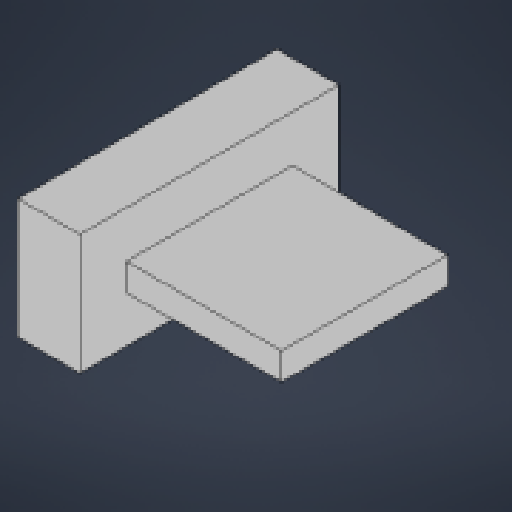
# Autodesk Inventor part: seguro1
Saved by Autodesk Inventor 2026.2 (Build 302298010, 298A)
## iProperties
Created: 2026-08-22
Part Number: seguro1
Material: Genérico
Document SubType Name: Modeling
Designer: samue
Density: 1 g/cm^3
Appearance: Valor por defecto
Author: samue
Autodesk Inventor part; units mm, degrees
ref_plane "YZ Plane" through (0, 0, 0) normal (1, 0, 0) x (0, 1, 0)
ref_plane "XZ Plane" through (0, 0, 0) normal (0, 1, 0) x (-1, 0, 0)
ref_plane "XY Plane" through (0, 0, 0) normal (0, 0, 1) x (1, 0, 0)
sketch "Boceto1" plane through (0, 0, 0) normal (1, 0, 0) x (0, 1, 0)
  line L0 (0, 0) -> (1.75, 0)
  line L1 (1.75, 0) -> (1.75, -10.7)
  line L2 (1.75, -10.7) -> (0, -10.7)
  line L3 (0, -10.7) -> (0, 0)
  dimension "d0" = 1.75
  dimension "d1" = 10.7
  constraints: 8 end point, 2 parallel, 1 horizontal, 1 perpendicular
  measures "d0" distance of L1.end L2.end
  measures "d1" distance of L0.end L1.end
extrude "Extrusión1" add sketch "Boceto1" along normal blind 10
sketch "Boceto2" plane through (0, 0, 0) normal (-1, 0, 0) x (0, 0, 1)
  line L0 (-10.7, 0) -> (-10.7, 1.75) projected
  line L1 (0, 0) -> (-10.7, 0) projected
  line L2 (0, 1.75) -> (0, 0) projected
  line L3 (-10.7, 1.75) -> (0, 1.75) projected
  line L4 (-13.7, -3) -> (-13.7, 4.75)
  line L5 (-13.7, 4.75) -> (3, 4.75)
  line L6 (3, 4.75) -> (3, -3)
  line L7 (3, -3) -> (-13.7, -3)
  dimension "d4" = 3
  constraints: 8 end point, 3 other
  measures "d4" distance between parallel lines of L1 L7
extrude "Extrusión2" add sketch "Boceto2" along normal blind 4 contours L0 L3 L2 L1 | L4 L5 L6 L7
